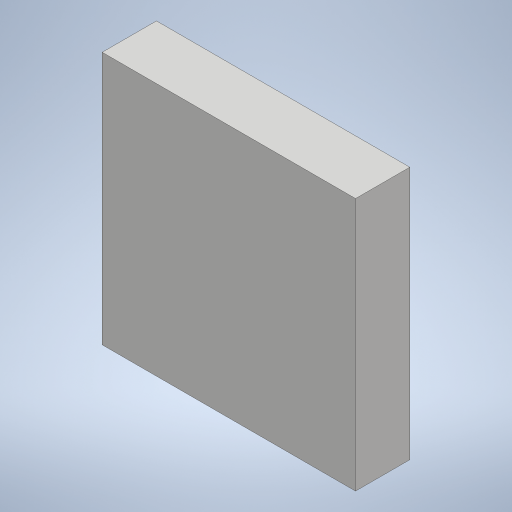
# Autodesk Inventor part: mordaza
Saved by Autodesk Inventor 2024.2 (Build 282272000, 272)
## iProperties
Created: 2025-06-19
Part Number: mordaza
Material: Genérico
Document SubType Name: Modeling
Designer: jd.castellanosq
Density: 1 g/cm^3
Appearance: Valor por defecto
Author: jd.castellanosq
Autodesk Inventor part; units mm, degrees
ref_plane "YZ Plane" through (0, 0, 0) normal (1, 0, 0) x (0, 1, 0)
ref_plane "XZ Plane" through (0, 0, 0) normal (0, 1, 0) x (-1, 0, 0)
ref_plane "XY Plane" through (0, 0, 0) normal (0, 0, 1) x (1, 0, 0)
sketch "Boceto1" plane through (0, 0, 0) normal (0, 1, 0) x (-1, 0, 0)
  line L0 (14, -14) -> (-14, -14)
  line L1 (-14, -14) -> (-14, 14)
  line L2 (-14, 14) -> (14, 14)
  line L3 (14, 14) -> (14, -14)
  point P0 (0, 0)
  point P1 (0, -14)
  point P2 (-14, 0)
  dimension "d0" = 28
  constraints: 8 end point, 2 midpoint, 2 parallel, 2 perpendicular, 1 horizontal, 1 horizontal alignment, 1 vertical alignment
  measures "d0" distance of L0.start L0.end
extrude "Extrusión1" add sketch "Boceto1" along normal blind 6
sketch "Boceto2" plane through (0, 6, 0) normal (0, 1, 0) x (1, 0, 0)
  circle A0 centre (0, 0) radius 2.5
  dimension "d3" = 5
  constraints: 1 centre point, 1 coincident
  measures "d3" diameter of A0
extrude "Extrusión2" cut sketch "Boceto2" against normal blind 5
sketch "Boceto3" plane through (14, 0, -14) normal (0, 0, -1) x (-1, 0, 0)
  line L0 (0, 0) -> (28, 0) projected
  line L1 (28, 0) -> (28, 6) projected
  point P0 (14, 0)
  point P1 (14, 3)
  point P2 (14, 0)
  point P3 (28, 3)
  constraints: 2 midpoint, 1 horizontal alignment, 1 vertical alignment
hole "Agujero1" at (0, 3, -14) direction (0, 0, 1) diameter 2.459 depth 14 tip angle 118 thread size "M3x0.5" class "6H" standard "ANSI Metric M Profile"
